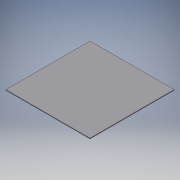
# Autodesk Inventor part: heated bed
Saved by Autodesk Inventor 2016 SP1 (Build 200210100, 210)
## iProperties
Created: 2016-04-14
Part Number: heated bed
Material: Generic
Document SubType Name: Modeling
Designer: ubik
Density: 1 g/cm^3
Appearance: Default
Author: ubik
Autodesk Inventor part; units mm, degrees
ref_plane "YZ Plane" through (0, 0, 0) normal (1, 0, 0) x (0, 1, 0)
ref_plane "XZ Plane" through (0, 0, 0) normal (0, 1, 0) x (-1, 0, 0)
ref_plane "XY Plane" through (0, 0, 0) normal (0, 0, 1) x (1, 0, 0)
sketch "Sketch1" plane through (0, 0, 0) normal (0, 0, 1) x (1, 0, 0)
  line L0 (107.5, 26.3211) -> (-107.5, 26.3211)
  line L1 (-107.5, 26.3211) -> (-107.5, 241.3211)
  line L2 (-107.5, 241.3211) -> (107.5, 241.3211)
  line L3 (107.5, 241.3211) -> (107.5, 26.3211)
  point P0 (0, 0)
  point P1 (0, 133.8211)
  dimension "d0" = 215
  dimension "d1" = 215
  dimension "d2" = 107.5
  dimension "d3" = 107.5
  constraints: 8 end point, 2 parallel, 1 horizontal, 1 perpendicular, 1 other
  measures "d0" distance of L0.start L0.end
  measures "d1" distance of L0.end L1.end
  measures "d2" distance from line of point (0, 133.821) L0
  measures "d3" distance from line of point (0, 133.821) L3
extrude "Extrusion1" add sketch "Sketch1" along normal blind 2
equation "\"d1\" = d0"
equation "\"d2\" = 0.5 * d1"
equation "\"d3\" = 0.5 * d0"
body "Solid1"
